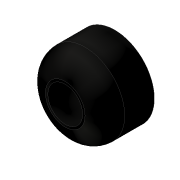
# Autodesk Inventor part: Feet
Saved by Autodesk Inventor 2017 (Build 210142000, 142)
## iProperties
Created: 2017-01-02
Part Number: Feet
Material: Generic
Document SubType Name: Modeling
Designer: ge937963
Density: 1 g/cm^3
Appearance: Smooth - Black
Author: ge937963
Autodesk Inventor part; units mm, degrees
ref_plane "YZ Plane" through (0, 0, 0) normal (1, 0, 0) x (0, 1, 0)
ref_plane "XZ Plane" through (0, 0, 0) normal (0, 1, 0) x (-1, 0, 0)
ref_plane "XY Plane" through (0, 0, 0) normal (0, 0, 1) x (1, 0, 0)
sketch "Sketch1" plane through (0, 0, 0) normal (0, 1, 0) x (-1, 0, 0)
  line L0 (0, 0) -> (5.08, 0)
  line L1 (5.08, 0) -> (5.08, 3.81)
  line L2 (2.54, 6.35) -> (0, 6.35)
  line L3 (0, 6.35) -> (0, 0)
  arc A0 (5.08, 3.81) -> (2.54, 6.35) centre (2.54, 3.81) ccw
  line L4 (1.5875, 0) -> (1.5875, 1.27)
  line L5 (1.5875, 1.27) -> (2.2294, 1.27)
  line L6 (2.2294, 1.27) -> (2.2294, 6.35)
  dimension "d0" = 2.54
  dimension "d1" = 5.08
  dimension "d2" = 6.35
  dimension "d3" = 1.5875
  dimension "d5" = 1.27
  constraints: 14 end point, 3 perpendicular, 2 parallel, 2 point on circle, 2 point on line, 2 tangent, 1 centre point, 1 horizontal, 1 vertical
  measures "d0" radius of A0
  measures "d1" distance of L0.start L0.end
  measures "d2" distance between parallel lines of L0 L2
  measures "d3" distance between parallel lines of L3 L4
  measures "d5" distance of L4.start L4.end
revolve "Revolution1" add sketch "Sketch1" angle 360 about axis through (0, 0, 6.35) along (0, 0, -1) contours L4 L5 L6 L2 A0 L1 L0
body "Solid1"
